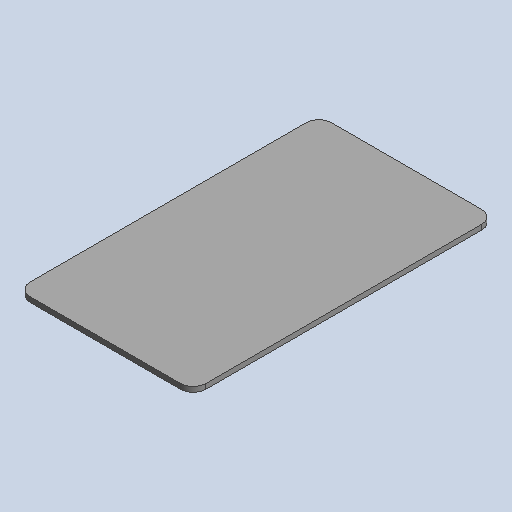
# Autodesk Inventor part: Enclosure_7
Saved by Autodesk Inventor 2026 (Build 300175050, 175E)
## iProperties
Part Number: Enclosure_7
Material: Generic
Document SubType Name: Modeling
Designer: Kartik
Mass: 134.057 g
Surface Area: 699.996 cm^2
Volume: 134.057 cm^3
Density: 1 g/cm^3
Appearance: Default
Author: Kartik
Autodesk Inventor part; units mm, degrees
ref_plane "YZ Plane" through (0, 0, 0) normal (1, 0, 0) x (0, 1, 0)
ref_plane "XZ Plane" through (0, 0, 0) normal (0, 1, 0) x (-1, 0, 0)
ref_plane "XY Plane" through (0, 0, 0) normal (0, 0, 1) x (1, 0, 0)
sketch "Sketch1" plane through (0, 0, 0) normal (0, 1, 0) x (-1, 0, 0)
  line L0 (68.019, 107.8294) -> (-71.981, 107.8294)
  line L1 (-71.981, 107.8294) -> (-71.981, -132.1706)
  line L2 (-71.981, -132.1706) -> (68.019, -132.1706)
  line L3 (68.019, -132.1706) -> (68.019, 107.8294)
  point P0 (0, 0)
  dimension "d0" = 240
  dimension "d1" = 140
  constraints: 8 end point, 2 parallel, 1 horizontal, 1 perpendicular
  measures "d0" distance of L2.end L0.start
  measures "d1" distance of L0.start L0.end
extrude "Extrusion1" add sketch "Sketch1" along normal blind 4
fillet "Fillet1" radius 10 4 edges at (71.981, 2, 107.8294) (-68.019, 2, 107.8294) (71.981, 2, -132.1706) (-68.019, 2, -132.1706)
body "Solid1"
